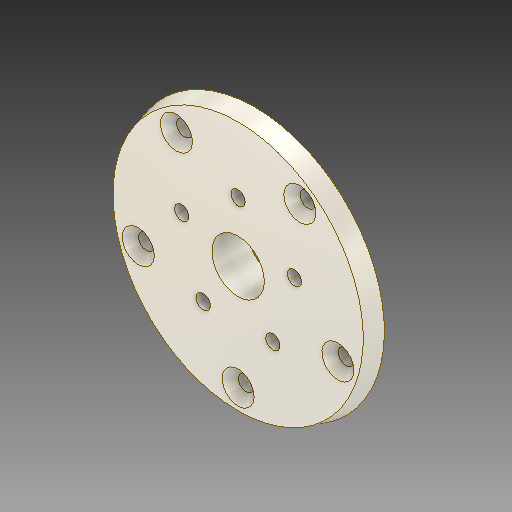
# Autodesk Inventor part: 332-01
Saved by Autodesk Inventor 2019 (Build 230136000, 136)
## iProperties
Company: Autodesk Inc.
Created: 2017-03-16
Part Number: 332-01
Material: Titanium
Document SubType Name: Modeling
Designer: Autodesk Inc.
Density: 4.51 g/cm^3
Appearance: Titanium
Mass: 369.113 g
Surface Area: 236.949 cm^2
Volume: 81.8433 cm^3
Author: Inventor
Autodesk Inventor part; units mm, degrees
ref_plane "YZ Plane" through (0, 0, 0) normal (1, 0, 0) x (0, 1, 0)
ref_plane "XZ Plane" through (0, 0, 0) normal (0, 1, 0) x (-1, 0, 0)
ref_plane "XY Plane" through (0, 0, 0) normal (0, 0, 1) x (1, 0, 0)
sketch "Sketch1" plane through (0, 0, 0) normal (0, 0, 1) x (1, 0, 0)
  circle A0 centre (0, 0) radius 11
  circle A1 centre (0, 0) radius 54.2995
  dimension "d0" = 22
  dimension "d1" = 108.599
  constraints: 2 centre point, 2 coincident
  measures "d0" diameter of A0
  measures "d1" diameter of A1
extrude "Extrusion1" add sketch "Sketch1" along normal blind 7
sketch "Sketch2" plane through (0, 0, 0) normal (0, 0, -1) x (-1, 0, 0)
  circle A0 centre (0, 0) radius 11 projected
  circle A1 centre (0, 0) radius 54.2995 projected
  circle A2 centre (0, 0) radius 34
  dimension "d4" = 68
  constraints: 1 centre point, 1 coincident
  measures "d4" diameter of A2
extrude "Extrusion2" add sketch "Sketch2" along normal blind 8 contours A2
sketch "Sketch3" plane through (0, 0, -8) normal (0, 0, -1) x (-1, 0, 0)
  circle A0 centre (0, 0) radius 11 projected
  point P0 (0, 24.84)
  dimension "d7" = 24.84
  constraints: 1 vertical alignment
  measures "d7" distance of A0.centre point (0, 24.84)
hole "Hole1" at (0, 24.84, -8) direction (0, 0, 1) diameter 6 end through all
sketch "Sketch4" plane through (0, 0, 7) normal (0, 0, 1) x (1, 0, 0)
  circle A0 centre (0, 0) radius 11 projected
  point P0 (0, -44)
  dimension "d15" = 44
  constraints: 1 vertical alignment
  measures "d15" distance of A0.centre point (0, -44)
hole "Hole2" at (0, -44, 7) direction (0, 0, -1) diameter 6.6 end through all countersink diameter 13.44 countersink angle 90
pattern_circular "Circular Pattern1" count 5 over 360 about axis through (0, 0, -10) along (0, 0, 1) of "Hole2", "Hole1"
sketch "Sketch5" plane through (0, 0, 0) normal (1, 0, 0) x (0, 1, 0)
  line L0 (21.84, 7) -> (21.84, -8) projected
  line L1 (21.84, -8) -> (11, -8) projected
  line L2 (11, -8) -> (11, 7) projected
  line L3 (11, 7) -> (21.84, 7) projected
  line L4 (-34, -8) -> (-34, 0) projected
  line L5 (-34, 0) -> (-40.7, 0) projected
  line L6 (-40.7, 0) -> (-40.7, 3.58) projected
  line L7 (-40.7, 3.58) -> (-37.28, 7) projected
  line L8 (-37.28, 7) -> (-11, 7) projected
  line L9 (-11, 7) -> (-11, -8) projected
  line L10 (-11, -8) -> (-34, -8) projected
  line L11 (-54.2995, 0) -> (-54.2995, 7) projected
  line L12 (-54.2995, 7) -> (-50.72, 7) projected
  line L13 (-50.72, 7) -> (-47.3, 3.58) projected
  line L14 (-47.3, 3.58) -> (-47.3, 0) projected
  line L15 (-47.3, 0) -> (-54.2995, 0) projected
  line L16 (54.2995, 7) -> (54.2995, 0) projected
  line L17 (54.2995, 0) -> (34, 0) projected
  line L18 (34, 0) -> (34, -8) projected
  line L19 (34, -8) -> (27.84, -8) projected
  line L20 (27.84, -8) -> (27.84, 7) projected
  line L21 (27.84, 7) -> (54.2995, 7) projected
  line L22 (54.2995, 0) -> (52.4239, 7)
  line L23 (0, -11) -> (0, 10) projected
  dimension "d26" = 15
  constraints: 2 end point, 1 point on line
  measures "d26" angle of L16 L22
revolve "Revolution1" cut sketch "Sketch5" angle 360 about axis through (0, 0, -10) along (0, 0, 1) contours L16 L22 L21
body "Solid1"
